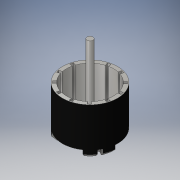
# Autodesk Inventor part: BrushlessOuter
Saved by Autodesk Inventor 2016 (Build 200138000, 138)
## iProperties
Created: 2016-02-03
Part Number: BrushlessOuter
Material: Generic
Document SubType Name: Modeling
Designer: Willis
Density: 1 g/cm^3
Appearance: Aluminum - Polished
Author: Willis
Autodesk Inventor part; units mm, degrees
ref_plane "YZ Plane" through (0, 0, 0) normal (1, 0, 0) x (0, 1, 0)
ref_plane "XZ Plane" through (0, 0, 0) normal (0, 1, 0) x (-1, 0, 0)
ref_plane "XY Plane" through (0, 0, 0) normal (0, 0, 1) x (1, 0, 0)
sketch "Sketch1" plane through (0, 0, 0) normal (0, 1, 0) x (-1, 0, 0)
  circle A0 centre (0, 0) radius 14
  arc A1 (11.7156, -2.5973) -> (11.7795, 2.2897) centre (0, 0) ccw
  line L0 (11.7156, -2.5973) -> (13.18, -2.9219)
  line L1 (13.252, 2.5759) -> (11.7795, 2.2897)
  line L2 (0, 0) -> (39.8589, 0) construction
  line L3 (11.7156, -2.5973) -> (0, 0) construction
  line L4 (11.7795, 2.2897) -> (0, 0) construction
  circle A2 centre (0, 0) radius 13.5
  arc A3 (11.4446, 3.6085) -> (9.0565, 7.8727) centre (0, 0) ccw
  line L5 (11.4446, 3.6085) -> (12.8752, 4.0595)
  line L6 (10.1886, 8.8568) -> (9.0565, 7.8727)
  arc A4 (8.1071, 8.8473) -> (3.9068, 11.3462) centre (0, 0) ccw
  line L7 (8.1071, 8.8473) -> (9.1205, 9.9532)
  line L8 (4.3952, 12.7645) -> (3.9068, 11.3462)
  arc A5 (2.5973, 11.7156) -> (-2.2897, 11.7795) centre (0, 0) ccw
  line L9 (2.5973, 11.7156) -> (2.9219, 13.18)
  line L10 (-2.5759, 13.252) -> (-2.2897, 11.7795)
  arc A6 (-3.6085, 11.4446) -> (-7.8727, 9.0565) centre (0, 0) ccw
  line L11 (-3.6085, 11.4446) -> (-4.0595, 12.8752)
  line L12 (-8.8568, 10.1886) -> (-7.8727, 9.0565)
  arc A7 (-8.8473, 8.1071) -> (-11.3462, 3.9068) centre (0, 0) ccw
  line L13 (-8.8473, 8.1071) -> (-9.9532, 9.1205)
  line L14 (-12.7645, 4.3952) -> (-11.3462, 3.9068)
  arc A8 (-11.7156, 2.5973) -> (-11.7795, -2.2897) centre (0, 0) ccw
  line L15 (-11.7156, 2.5973) -> (-13.18, 2.9219)
  line L16 (-13.252, -2.5759) -> (-11.7795, -2.2897)
  arc A9 (-11.4446, -3.6085) -> (-9.0565, -7.8727) centre (0, 0) ccw
  line L17 (-11.4446, -3.6085) -> (-12.8752, -4.0595)
  line L18 (-10.1886, -8.8568) -> (-9.0565, -7.8727)
  arc A10 (-8.1071, -8.8473) -> (-3.9068, -11.3462) centre (0, 0) ccw
  line L19 (-8.1071, -8.8473) -> (-9.1205, -9.9532)
  line L20 (-4.3952, -12.7645) -> (-3.9068, -11.3462)
  arc A11 (-2.5973, -11.7156) -> (2.2897, -11.7795) centre (0, 0) ccw
  line L21 (-2.5973, -11.7156) -> (-2.9219, -13.18)
  line L22 (2.5759, -13.252) -> (2.2897, -11.7795)
  arc A12 (3.6085, -11.4446) -> (7.8727, -9.0565) centre (0, 0) ccw
  line L23 (3.6085, -11.4446) -> (4.0595, -12.8752)
  line L24 (8.8568, -10.1886) -> (7.8727, -9.0565)
  arc A13 (8.8473, -8.1071) -> (11.3462, -3.9068) centre (0, 0) ccw
  line L25 (8.8473, -8.1071) -> (9.9532, -9.1205)
  line L26 (12.7645, -4.3952) -> (11.3462, -3.9068)
  dimension "d0" = 28
  dimension "d1" = 2
  dimension "d2" = 23.5
  dimension "d4" = 12.5
  dimension "d5" = 12.5
  dimension "d6" = 0.5
  dimension "d9" = 360
  constraints: 54 end point, 26 point on circle, 14 centre point, 3 coincident, 1 collinear, 1 horizontal, 97 other
  measures "d0" diameter of A0
  measures "d1" radial gap between concentric circles of A0 A1
  measures "d2" angle of L0 L1
  measures "d4" angle of L2 L0
  measures "d5" angle of L2 L3
  measures "d6" radial gap between concentric circles of A0 A2
extrude "Extrusion1" add sketch "Sketch1" along normal blind 20
sketch "Sketch2" plane through (0, 0, 0) normal (0, 1, 0) x (-1, 0, 0)
  circle A0 centre (0, 0) radius 14
  arc A1 (11.7156, -2.5973) -> (11.7795, 2.2897) centre (0, 0) ccw
  line L0 (11.7156, -2.5973) -> (13.18, -2.9219)
  line L1 (13.252, 2.5759) -> (11.7795, 2.2897)
  line L2 (0, 0) -> (39.8589, 0) construction
  line L3 (11.7156, -2.5973) -> (0, 0) construction
  line L4 (11.7795, 2.2897) -> (0, 0) construction
  circle A2 centre (0, 0) radius 13.5
  arc A3 (11.4446, 3.6085) -> (9.0565, 7.8727) centre (0, 0) ccw
  line L5 (11.4446, 3.6085) -> (12.8752, 4.0595)
  line L6 (10.1886, 8.8568) -> (9.0565, 7.8727)
  arc A4 (8.1071, 8.8473) -> (3.9068, 11.3462) centre (0, 0) ccw
  line L7 (8.1071, 8.8473) -> (9.1205, 9.9532)
  line L8 (4.3952, 12.7645) -> (3.9068, 11.3462)
  arc A5 (2.5973, 11.7156) -> (-2.2897, 11.7795) centre (0, 0) ccw
  line L9 (2.5973, 11.7156) -> (2.9219, 13.18)
  line L10 (-2.5759, 13.252) -> (-2.2897, 11.7795)
  arc A6 (-3.6085, 11.4446) -> (-7.8727, 9.0565) centre (0, 0) ccw
  line L11 (-3.6085, 11.4446) -> (-4.0595, 12.8752)
  line L12 (-8.8568, 10.1886) -> (-7.8727, 9.0565)
  arc A7 (-8.8473, 8.1071) -> (-11.3462, 3.9068) centre (0, 0) ccw
  line L13 (-8.8473, 8.1071) -> (-9.9532, 9.1205)
  line L14 (-12.7645, 4.3952) -> (-11.3462, 3.9068)
  arc A8 (-11.7156, 2.5973) -> (-11.7795, -2.2897) centre (0, 0) ccw
  line L15 (-11.7156, 2.5973) -> (-13.18, 2.9219)
  line L16 (-13.252, -2.5759) -> (-11.7795, -2.2897)
  arc A9 (-11.4446, -3.6085) -> (-9.0565, -7.8727) centre (0, 0) ccw
  line L17 (-11.4446, -3.6085) -> (-12.8752, -4.0595)
  line L18 (-10.1886, -8.8568) -> (-9.0565, -7.8727)
  arc A10 (-8.1071, -8.8473) -> (-3.9068, -11.3462) centre (0, 0) ccw
  line L19 (-8.1071, -8.8473) -> (-9.1205, -9.9532)
  line L20 (-4.3952, -12.7645) -> (-3.9068, -11.3462)
  arc A11 (-2.5973, -11.7156) -> (2.2897, -11.7795) centre (0, 0) ccw
  line L21 (-2.5973, -11.7156) -> (-2.9219, -13.18)
  line L22 (2.5759, -13.252) -> (2.2897, -11.7795)
  arc A12 (3.6085, -11.4446) -> (7.8727, -9.0565) centre (0, 0) ccw
  line L23 (3.6085, -11.4446) -> (4.0595, -12.8752)
  line L24 (8.8568, -10.1886) -> (7.8727, -9.0565)
  arc A13 (8.8473, -8.1071) -> (11.3462, -3.9068) centre (0, 0) ccw
  line L25 (8.8473, -8.1071) -> (9.9532, -9.1205)
  line L26 (12.7645, -4.3952) -> (11.3462, -3.9068)
  dimension "d15" = 28
  dimension "d16" = 2
  dimension "d17" = 23.5
  dimension "d18" = 12.5
  dimension "d19" = 12.5
  dimension "d20" = 0.5
  dimension "d21" = 360
  constraints: 54 end point, 26 point on circle, 14 centre point, 3 coincident, 1 collinear, 1 horizontal, 97 other
  measures "d15" diameter of A0
  measures "d16" radial gap between concentric circles of A0 A1
  measures "d17" angle of L0 L1
  measures "d18" angle of L2 L0
  measures "d19" angle of L2 L3
  measures "d20" radial gap between concentric circles of A0 A2
extrude "Extrusion2" add sketch "Sketch2" along normal blind 20 contours A1 L1 A2 L0
pattern_circular "Circular Pattern1" count 12 over 360 about axis through (0, 0, 0) along (0, 1, 0) of "Extrusion2"
sketch "Sketch3" plane through (0, 0, 0) normal (0, -1, 0) x (1, 0, 0)
  circle A0 centre (0, 0) radius 14
  circle A1 centre (0, 0) radius 12
  dimension "d27" = 28
  dimension "d28" = 24
  constraints: 2 centre point, 2 coincident
  measures "d27" diameter of A0
  measures "d28" diameter of A1
extrude "Extrusion3" add sketch "Sketch3" against normal blind 4
sketch "Sketch4" plane through (0, 0, 0) normal (0, -1, 0) x (1, 0, 0)
  circle A0 centre (0, 0) radius 4.5
  line L0 (0, 0) -> (6, -12.6491)
  line L1 (0, 0) -> (-6, -12.6491)
  line L2 (0, 0) -> (0, -12.6491) construction
  line L3 (0, -12.6491) -> (6, -12.6491) construction
  line L4 (0, -12.6491) -> (-6, -12.6491) construction
  line L5 (0, 0) -> (0, -29.857) construction
  arc A1 (-6, -12.6491) -> (6, -12.6491) centre (0, 0) ccw
  dimension "d37" = 9
  dimension "d38" = 12
  dimension "d40" = 28
  constraints: 12 end point, 2 centre point, 2 coincident, 2 collinear, 2 point on circle, 2 vertical
  measures "d37" diameter of A0
  measures "d38" distance of L0.end L1.end
  measures "d40" diameter of A1
extrude "Extrusion4" add sketch "Sketch4" along normal blind 4
fillet "Fillet1" radius 2 2 edges at (-1.9286, -2, -4.0658) (1.9286, -2, -4.0658)
chamfer "Chamfer1" distance 2 angle 45 1 edges at (0, -4, -14)
pattern_circular "Circular Pattern2" count 3 over 360 about axis through (0, 0, 0) along (0, 1, 0) of "Extrusion4", "Chamfer1", "Fillet1"
sketch "Sketch5" plane through (0, -4, 0) normal (0, -1, 0) x (1, 0, 0)
  circle A0 centre (0, 0) radius 4
  dimension "d50" = 8
  constraints: 1 centre point, 1 coincident
  measures "d50" diameter of A0
extrude "Extrusion5" add sketch "Sketch5" along normal blind 2
sketch "Sketch6" plane through (0, -6, 0) normal (0, -1, 0) x (1, 0, 0)
  circle A0 centre (0, 0) radius 1.5
  dimension "d53" = 3
  constraints: 1 centre point, 1 coincident
  measures "d53" diameter of A0
extrude "Extrusion6" cut sketch "Sketch6" against normal blind 0.25
sketch "Sketch7" plane through (0, -5.75, 0) normal (0, -1, 0) x (1, 0, 0)
  circle A0 centre (0, 0) radius 1.5
  constraints: 1 centre point, 1 coincident
extrude "Extrusion7" add sketch "Sketch7" against normal blind 45
fillet "Fillet2" radius 0.5 1 edges at (-4, -6, 0)
sketch "Sketch8" plane through (0, -4, 0) normal (0, -1, 0) x (1, 0, 0)
  circle A0 centre (0, 0) radius 1.5 projected
  line L0 (0, 0) -> (5.5, 3.1754) construction
  line L1 (5.5, 3.1754) -> (-5.5, 3.1754) construction
  line L2 (-5.5, 3.1754) -> (0, -6.3509) construction
  line L3 (0, -6.3509) -> (5.5, 3.1754) construction
  line L4 (0, -6.3509) -> (0, 0) construction
  line L5 (-5.5, 3.1754) -> (0, 0) construction
  circle A1 centre (0, -6.3509) radius 1 construction
  circle A2 centre (5.5, 3.1754) radius 1
  circle A3 centre (-5.5, 3.1754) radius 1 construction
  line L6 (5.5, 3.1754) -> (8.9641, 5.1754) construction
  arc A4 (8.4641, 6.0415) -> (9.4641, 4.3094) centre (8.9641, 5.1754) ccw
  line L7 (8.4641, 6.0415) -> (11.5934, 7.8481)
  arc A5 (13.9545, 1.1284) -> (7.9545, 11.5207) centre (0, 0) ccw projected
  line L8 (9.4641, 4.3094) -> (12.5934, 6.1161)
  dimension "d59" = 2
  dimension "d60" = 11
  dimension "d61" = 4
  dimension "d62" = 2
  dimension "d63" = 2
  constraints: 18 end point, 4 centre point, 4 coincident, 4 equal length, 4 point on circle, 2 equal radius, 1 collinear, 1 horizontal, 1 parallel, 1 perpendicular, 1 tangent
  measures "d59" diameter of A3
  measures "d60" distance of L0.end L1.end
  measures "d61" distance of L6.start L6.end
  measures "d62" diameter of A4
  measures "d63" distance between parallel lines of L7 L8
extrude "Extrusion8" cut sketch "Sketch8" against normal up to surface (4 mm away) contours A2 | L7 A5 L8 A4
pattern_circular "Circular Pattern3" count 3 over 360 about axis through (0, 0, 0) along (0, 1, 0) of "Extrusion8"
body "Solid1"
